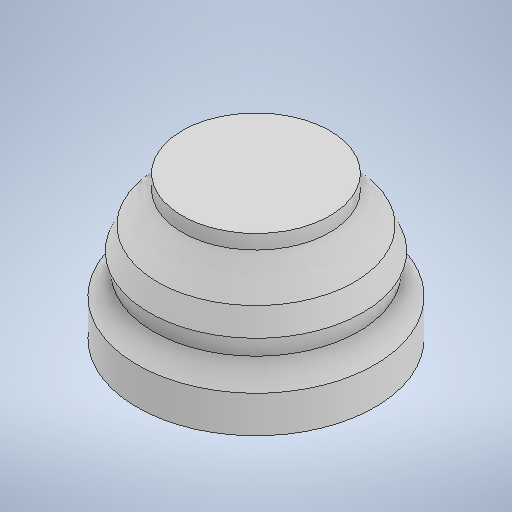
# Autodesk Inventor part: KINGHT BASE 1.1
Saved by Autodesk Inventor 2025.1 (Build 291241000, 241)
## iProperties
Created: 2024-10-24
Part Number: KINGHT BASE 1.1
Material: Genérico
Document SubType Name: Modeling
Designer: Octavio
Density: 1 g/cm^3
Appearance: Valor por defecto
Author: Octavio
Autodesk Inventor part; units mm, degrees
ref_plane "YZ Plane" through (0, 0, 0) normal (1, 0, 0) x (0, 1, 0)
ref_plane "XZ Plane" through (0, 0, 0) normal (0, 1, 0) x (-1, 0, 0)
ref_plane "XY Plane" through (0, 0, 0) normal (0, 0, 1) x (1, 0, 0)
sketch "Boceto2" plane through (0, 0, 0) normal (0, 0, 1) x (1, 0, 0)
  line L0 (-105.6698, 187.1112) -> (110.1141, 187.1112) construction
  line L1 (110.1141, 187.1112) -> (110.1141, -25.0762) construction
  line L2 (110.1141, -25.0762) -> (-105.6698, -25.0762) construction
  line L3 (-105.6698, -25.0762) -> (-105.6698, 187.1112) construction
  line L4 (0, 0) -> (0, 52.867)
  line L5 (0, 52.867) -> (0, 0)
  line L6 (-43.8447, 1.5105) -> (-43.8447, 13.5944)
  line L7 (-43.8447, 13.5944) -> (-37.8028, 21.1468)
  line L8 (-37.8028, 21.1468) -> (-39.3133, 27.944)
  line L9 (-39.3133, 27.944) -> (-36.2923, 36.2517)
  line L10 (-36.2923, 36.2517) -> (-32.6671, 40.7831)
  line L11 (-32.6671, 40.7831) -> (-30.2503, 43.8041)
  line L12 (-30.2503, 43.8041) -> (-27.2294, 47.5803)
  line L13 (-27.2294, 47.5803) -> (-27.2294, 52.867)
  line L14 (-27.2294, 52.867) -> (-23, 52.867)
  line L15 (0, 52.867) -> (-23, 52.867)
  line L16 (-27.2294, 52.867) -> (-23, 52.867)
  line L17 (0, 0) -> (-43.8447, 0)
  line L18 (-43.8447, 0) -> (-43.8447, 1.5105)
  dimension "d18" = 23
  constraints: 30 end point, 3 point on line, 2 collinear, 2 horizontal, 2 parallel, 2 vertical, 1 perpendicular, 2 other
  measures "d18" distance of L14.end L4.end
revolve "Revolución1" add sketch "Boceto2" angle 360 about axis through (0, 0, 0) along (0, 1, 0)
